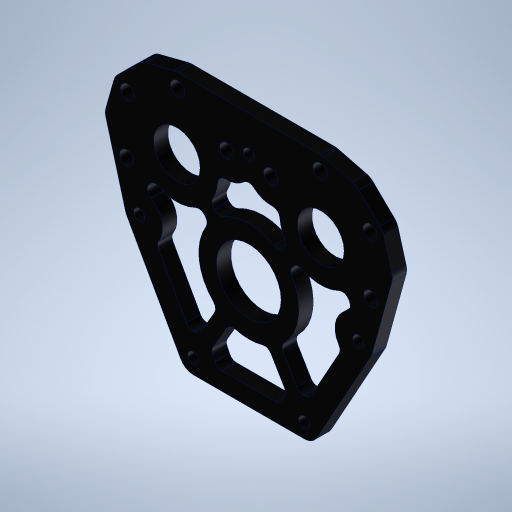
# Autodesk Inventor part: BottomPlate_Gearboxes_2_Exercise_2
Saved by Autodesk Inventor 2024 (Build 280153000, 153)
## iProperties
Created: 2024-11-16
Part Number: BottomPlate_Gearboxes_2_Exercise_2
Material: Aluminum 6061
Document SubType Name: Modeling
Designer: Danielle
Density: 2.7 g/cm^3
Appearance: Aluminum - Flat
Author: Danielle
Autodesk Inventor part; units mm, degrees
ref_plane "YZ Plane" through (0, 0, 0) normal (1, 0, 0) x (0, 1, 0)
ref_plane "XZ Plane" through (0, 0, 0) normal (0, 1, 0) x (-1, 0, 0)
ref_plane "XY Plane" through (0, 0, 0) normal (0, 0, 1) x (1, 0, 0)
sketch "Sketch1" plane through (0, 0, 0) normal (0, 0, 1) x (1, 0, 0)
  circle A0 centre (0, 0) radius 38.1 construction
  circle A1 centre (0, 0) radius 40.64 construction
  circle A2 centre (0, 0) radius 14.2875
  circle A3 centre (-31.9157, 32.7369) radius 30.0609 construction
  circle A4 centre (-31.9157, 32.7369) radius 25.4 construction
  circle A5 centre (-31.9157, 32.7369) radius 7.62 construction
  circle A6 centre (-53.7497, 45.7153) radius 3.175
  circle A7 centre (-57.3137, 33.0595) radius 3.175 construction
  circle A8 centre (-54.0723, 20.3173) radius 3.175
  circle A9 centre (-44.8941, 10.903) radius 3.175 construction
  circle A10 centre (-32.2383, 7.339) radius 3.175 construction
  circle A11 centre (-19.4961, 10.5803) radius 3.175 construction
  circle A12 centre (-10.0817, 19.7586) radius 3.175 construction
  circle A13 centre (-6.5178, 32.4143) radius 3.175 construction
  circle A14 centre (-9.7591, 45.1565) radius 3.175
  circle A15 centre (-18.9373, 54.5709) radius 3.175 construction
  circle A16 centre (-31.5931, 58.1349) radius 3.175
  circle A17 centre (-44.3353, 54.8935) radius 3.175 construction
  line L0 (-54.0723, 20.3173) -> (0, 0) construction
  line L1 (0, 0) -> (-18.9373, 54.5709) construction
  circle A18 centre (-48.5745, 1.2342) radius 2.4892
  circle A19 centre (-48.5745, 1.2342) radius 6.35 construction
  circle A20 centre (-48.5745, 1.2342) radius 3.9751 construction
  line L2 (-46.7163, 4.7482) -> (-45.9682, 6.1628) construction
  line L3 (-42.2266, 1.0729) -> (-40.6269, 1.0322) construction
  circle A21 centre (0, 48.5902) radius 6.35 construction
  circle A22 centre (0, 48.5902) radius 3.9751 construction
  circle A23 centre (0, 48.5902) radius 2.4892
  line L4 (0, 42.2402) -> (0, 40.64) construction
  line L5 (-3.5601, 46.8218) -> (-4.9932, 46.1099) construction
  circle A24 centre (-24.6505, -41.8731) radius 6.35 construction
  circle A25 centre (-24.6505, -41.8731) radius 2.4892
  line L6 (-21.4291, -36.4009) -> (-20.6173, -35.022)
  line L7 (0, 48.5902) -> (0, 0) construction
  circle A26 centre (31.9157, 32.7369) radius 30.0609 construction
  circle A27 centre (31.9157, 32.7369) radius 25.4 construction
  circle A28 centre (53.7497, 45.7153) radius 3.175
  circle A29 centre (57.3137, 33.0595) radius 3.175 construction
  circle A30 centre (54.0723, 20.3173) radius 3.175
  circle A31 centre (44.8941, 10.903) radius 3.175 construction
  circle A32 centre (9.7591, 45.1565) radius 3.175
  circle A33 centre (18.9373, 54.5709) radius 3.175 construction
  circle A34 centre (31.5931, 58.1349) radius 3.175
  circle A35 centre (44.3353, 54.8935) radius 3.175 construction
  circle A36 centre (48.5745, 1.2342) radius 2.4892
  circle A37 centre (48.5745, 1.2342) radius 6.35 construction
  circle A38 centre (48.5745, 1.2342) radius 3.9751 construction
  circle A39 centre (0, 48.5902) radius 2.4892 construction
  circle A40 centre (24.6505, -41.8731) radius 6.35 construction
  circle A41 centre (24.6505, -41.8731) radius 2.4892
  circle A42 centre (31.9157, 32.7369) radius 7.62 construction
  line L8 (-48.5745, 1.2342) -> (-24.6505, -41.8731) construction
  line L9 (24.6505, -41.8731) -> (-24.6505, -41.8731) construction
  circle A43 centre (-31.9157, 32.7369) radius 10.3188
  circle A44 centre (31.9157, 32.7369) radius 10.3188
  line L10 (-54.1268, -1.8472) -> (-30.2028, -44.9545)
  line L11 (-24.6505, -48.2231) -> (24.6505, -48.2231)
  line L12 (30.2028, -44.9545) -> (54.1268, -1.8472)
  circle A45 centre (44.3353, 54.8935) radius 6.35 construction
  circle A46 centre (53.7497, 45.7153) radius 6.35 construction
  circle A47 centre (31.5931, 58.1349) radius 6.35 construction
  circle A48 centre (57.3137, 33.0595) radius 6.35 construction
  circle A49 centre (54.0723, 20.3173) radius 6.35 construction
  circle A50 centre (-54.0723, 20.3173) radius 6.35 construction
  circle A51 centre (-57.3137, 33.0595) radius 6.35 construction
  circle A52 centre (-53.7497, 45.7153) radius 6.35 construction
  circle A53 centre (-44.3353, 54.8935) radius 6.35 construction
  circle A54 centre (-31.5931, 58.1349) radius 6.35 construction
  line L13 (-63.4259, 34.7808) -> (-59.8619, 47.4366)
  line L14 (-58.1824, 50.2621) -> (-48.768, 59.4403)
  line L15 (-45.9008, 61.0475) -> (-33.1586, 64.2889)
  line L16 (63.4259, 34.7808) -> (59.8619, 47.4366)
  line L17 (58.1824, 50.2621) -> (48.768, 59.4403)
  line L18 (45.9008, 61.0475) -> (33.1586, 64.2889)
  line L19 (-63.437, 31.3781) -> (-54.6979, -0.4473)
  line L20 (63.437, 31.3781) -> (54.6979, -0.4473)
  line L21 (-31.5931, 64.4849) -> (31.5931, 64.4849)
  arc A55 (-30.2028, -44.9545) -> (-24.6505, -48.2231) centre (-24.6505, -41.8731) ccw
  arc A56 (-54.6979, -0.4473) -> (-54.1268, -1.8472) centre (-48.5745, 1.2342) ccw
  arc A57 (-63.4259, 34.7808) -> (-63.437, 31.3781) centre (-57.3137, 33.0595) ccw
  arc A58 (-58.1824, 50.2621) -> (-59.8619, 47.4366) centre (-53.7497, 45.7153) ccw
  arc A59 (-45.9008, 61.0475) -> (-48.768, 59.4403) centre (-44.3353, 54.8935) ccw
  arc A60 (-31.5931, 64.4849) -> (-33.1586, 64.2889) centre (-31.5931, 58.1349) ccw
  arc A61 (33.1586, 64.2889) -> (31.5931, 64.4849) centre (31.5931, 58.1349) ccw
  arc A62 (48.768, 59.4403) -> (45.9008, 61.0475) centre (44.3353, 54.8935) ccw
  arc A63 (59.8619, 47.4366) -> (58.1824, 50.2621) centre (53.7497, 45.7153) ccw
  arc A64 (63.437, 31.3781) -> (63.4259, 34.7808) centre (57.3137, 33.0595) ccw
  arc A65 (54.1268, -1.8472) -> (54.6979, -0.4473) centre (48.5745, 1.2342) ccw
  arc A66 (24.6505, -48.2231) -> (30.2028, -44.9545) centre (24.6505, -41.8731) ccw
  dimension "d4" = 50.8
  dimension "d15" = 7.9502
  dimension "d22" = 12.7
  dimension "d0" = 76.2
  dimension "d1" = 2.54
  dimension "d2" = 28.575
  dimension "d3" = 60.1218
  dimension "d5" = 15.24
  dimension "d6" = 6.35
  dimension "d9" = 360
  dimension "d12" = 12.7
  dimension "d14" = 4.9784
  dimension "d16" = 1.6002
  dimension "d17" = 15.24
  dimension "d18" = 20.6375
  dimension "d19" = 20.6375
  dimension "d20" = 12.7
  dimension "d21" = 12.7
  dimension "d23" = 12.7
  dimension "d24" = 12.7
  dimension "d25" = 12.7
  dimension "d26" = 12.7
  dimension "d27" = 12.7
  dimension "d28" = 12.7
  dimension "d29" = 12.7
  constraints: 60 centre point, 45 point on circle, 44 end point, 25 coincident, 23 symmetric about line, 18 tangent, 10 point on line, 9 concentric, 6 equal length, 3 equal radius, 3 horizontal, 3 vertical, 2 vertical alignment, 63 other
  measures "d0" diameter of A0
  measures "d1" radial gap between concentric circles of A1 A0
  measures "d2" diameter of A2
  measures "d3" diameter of A3
  measures "d5" diameter of A5
  measures "d6" diameter of A6
  measures "d12" diameter of A19
  measures "d14" diameter of A18
  measures "d16" distance of L2.start L2.end
  measures "d17" diameter of A42
  measures "d18" diameter of A43
  measures "d19" diameter of A44
  measures "d20" diameter of A45
  measures "d21" diameter of A46
  measures "d23" diameter of A48
  measures "d24" diameter of A49
  measures "d25" diameter of A50
  measures "d26" diameter of A51
  measures "d27" diameter of A52
  measures "d28" diameter of A53
  measures "d29" diameter of A54
extrude "Extrusion1" add sketch "Sketch1" along normal blind 6.35
sketch "Sketch2" plane through (0, 0, 6.35) normal (0, 0, 1) x (1, 0, 0)
  line L0 (-63.437, 31.3781) -> (-54.6979, -0.4473) construction
  arc A0 (-54.6979, -0.4473) -> (-54.1268, -1.8472) centre (-48.5745, 1.2342) ccw construction
  line L1 (-54.1268, -1.8472) -> (-30.2028, -44.9545) construction
  arc A1 (-30.2028, -44.9545) -> (-24.6505, -48.2231) centre (-24.6505, -41.8731) ccw construction
  line L2 (-24.6505, -48.2231) -> (24.6505, -48.2231) construction
  arc A2 (24.6505, -48.2231) -> (30.2028, -44.9545) centre (24.6505, -41.8731) ccw construction
  line L3 (30.2028, -44.9545) -> (54.1268, -1.8472) construction
  arc A3 (54.1268, -1.8472) -> (54.6979, -0.4473) centre (48.5745, 1.2342) ccw construction
  line L4 (54.6979, -0.4473) -> (63.437, 31.3781) construction
  arc A4 (63.437, 31.3781) -> (63.4259, 34.7808) centre (57.3137, 33.0595) ccw construction
  line L5 (63.4259, 34.7808) -> (59.8619, 47.4366) construction
  arc A5 (59.8619, 47.4366) -> (58.1824, 50.2621) centre (53.7497, 45.7153) ccw construction
  line L6 (58.1824, 50.2621) -> (48.768, 59.4403) construction
  arc A6 (48.768, 59.4403) -> (45.9008, 61.0475) centre (44.3353, 54.8935) ccw construction
  line L7 (45.9008, 61.0475) -> (33.1586, 64.2889) construction
  arc A7 (33.1586, 64.2889) -> (31.5931, 64.4849) centre (31.5931, 58.1349) ccw construction
  line L8 (31.5931, 64.4849) -> (-31.5931, 64.4849) construction
  arc A8 (-31.5931, 64.4849) -> (-33.1586, 64.2889) centre (-31.5931, 58.1349) ccw construction
  line L9 (-33.1586, 64.2889) -> (-45.9008, 61.0475) construction
  arc A9 (-45.9008, 61.0475) -> (-48.768, 59.4403) centre (-44.3353, 54.8935) ccw construction
  line L10 (-48.768, 59.4403) -> (-58.1824, 50.2621) construction
  arc A10 (-58.1824, 50.2621) -> (-59.8619, 47.4366) centre (-53.7497, 45.7153) ccw construction
  line L11 (-59.8619, 47.4366) -> (-63.4259, 34.7808) construction
  arc A11 (-63.4259, 34.7808) -> (-63.437, 31.3781) centre (-57.3137, 33.0595) ccw construction
  circle A12 centre (31.9157, 32.7369) radius 10.3188 construction
  circle A13 centre (24.6505, -41.8731) radius 2.4892 construction
  circle A14 centre (9.7591, 45.1565) radius 3.175 construction
  circle A15 centre (53.7497, 45.7153) radius 3.175 construction
  circle A16 centre (0, 48.5902) radius 2.4892 construction
  circle A17 centre (-48.5745, 1.2342) radius 2.4892 construction
  circle A18 centre (-9.7591, 45.1565) radius 3.175 construction
  circle A19 centre (-53.7497, 45.7153) radius 3.175 construction
  circle A20 centre (0, 0) radius 14.2875 construction
  circle A21 centre (-24.6505, -41.8731) radius 2.4892 construction
  circle A22 centre (48.5745, 1.2342) radius 2.4892 construction
  circle A23 centre (-31.9157, 32.7369) radius 10.3188 construction
  circle A24 centre (31.5931, 58.1349) radius 3.175 construction
  circle A25 centre (54.0723, 20.3173) radius 3.175 construction
  circle A26 centre (-31.5931, 58.1349) radius 3.175 construction
  circle A27 centre (-54.0723, 20.3173) radius 3.175 construction
  circle A28 centre (-31.9157, 32.7369) radius 15.0813 construction
  circle A29 centre (31.9157, 32.7369) radius 15.0813 construction
  circle A30 centre (-31.5931, 58.1349) radius 7.9375 construction
  circle A31 centre (-53.7497, 45.7153) radius 7.9375 construction
  circle A32 centre (-54.0723, 20.3173) radius 7.9375 construction
  circle A33 centre (-9.7591, 45.1565) radius 7.9375 construction
  circle A34 centre (9.7591, 45.1565) radius 7.9375 construction
  circle A35 centre (31.5931, 58.1349) radius 7.9375 construction
  circle A36 centre (53.7497, 45.7153) radius 7.9375 construction
  circle A37 centre (54.0723, 20.3173) radius 7.9375 construction
  circle A38 centre (0, 48.5902) radius 7.2517 construction
  circle A39 centre (48.5745, 1.2342) radius 7.2517 construction
  circle A40 centre (24.6505, -41.8731) radius 7.2517 construction
  circle A41 centre (-24.6505, -41.8731) radius 7.2517 construction
  circle A42 centre (-48.5745, 1.2342) radius 7.2517 construction
  circle A43 centre (0, 0) radius 19.05 construction
  line L12 (-26.0386, -42.6435) -> (-49.9626, 0.4638) construction
  arc A44 (-50.1054, 0.8138) -> (-49.9626, 0.4638) centre (-48.5745, 1.2342) ccw construction
  line L13 (-50.1054, 0.8138) -> (-58.8445, 32.6392) construction
  arc A45 (-58.8417, 33.4898) -> (-58.8445, 32.6392) centre (-57.3137, 33.0595) ccw construction
  line L14 (-58.8417, 33.4898) -> (-55.2777, 46.1456) construction
  arc A46 (-54.8579, 46.852) -> (-55.2777, 46.1456) centre (-53.7497, 45.7153) ccw construction
  line L15 (-54.8579, 46.852) -> (-45.4435, 56.0302) construction
  arc A47 (-44.7267, 56.432) -> (-45.4435, 56.0302) centre (-44.3353, 54.8935) ccw construction
  line L16 (-44.7267, 56.432) -> (-31.9845, 59.6734) construction
  arc A48 (-31.5931, 59.7224) -> (-31.9845, 59.6734) centre (-31.5931, 58.1349) ccw construction
  line L17 (-31.5931, 59.7224) -> (31.5931, 59.7224) construction
  arc A49 (31.9845, 59.6734) -> (31.5931, 59.7224) centre (31.5931, 58.1349) ccw construction
  line L18 (31.9845, 59.6734) -> (44.7267, 56.432) construction
  arc A50 (45.4435, 56.0302) -> (44.7267, 56.432) centre (44.3353, 54.8935) ccw construction
  line L19 (45.4435, 56.0302) -> (54.8579, 46.852) construction
  arc A51 (55.2777, 46.1456) -> (54.8579, 46.852) centre (53.7497, 45.7153) ccw construction
  line L20 (55.2777, 46.1456) -> (58.8417, 33.4898) construction
  arc A52 (58.8445, 32.6392) -> (58.8417, 33.4898) centre (57.3137, 33.0595) ccw construction
  line L21 (58.8445, 32.6392) -> (50.1054, 0.8138) construction
  arc A53 (49.9626, 0.4638) -> (50.1054, 0.8138) centre (48.5745, 1.2342) ccw construction
  line L22 (49.9626, 0.4638) -> (26.0386, -42.6435) construction
  arc A54 (24.6505, -43.4606) -> (26.0386, -42.6435) centre (24.6505, -41.8731) ccw construction
  line L23 (24.6505, -43.4606) -> (-24.6505, -43.4606) construction
  arc A55 (-26.0386, -42.6435) -> (-24.6505, -43.4606) centre (-24.6505, -41.8731) ccw construction
  line L24 (-53.7497, 45.7153) -> (-31.9157, 32.7369) construction
  line L25 (-31.9157, 32.7369) -> (0, 0) construction
  line L26 (0, 0) -> (24.6505, -41.8731) construction
  line L27 (-31.5931, 58.1349) -> (-9.7591, 45.1565) construction
  line L28 (-9.7591, 45.1565) -> (0, 48.5902) construction
  line L29 (0, 48.5902) -> (9.7591, 45.1565) construction
  line L30 (9.7591, 45.1565) -> (31.9157, 32.7369) construction
  line L31 (31.9157, 32.7369) -> (53.7497, 45.7153) construction
  line L32 (9.7591, 45.1565) -> (31.5931, 58.1349) construction
  line L33 (31.9157, 32.7369) -> (54.0723, 20.3173) construction
  line L34 (31.9157, 32.7369) -> (0, 0) construction
  line L35 (-24.6505, -41.8731) -> (0, 0) construction
  line L36 (-53.7497, 45.7153) -> (-54.0723, 20.3173) construction
  line L37 (-54.0723, 20.3173) -> (-31.9157, 32.7369) construction
  line L38 (-31.9157, 32.7369) -> (-9.7591, 45.1565) construction
  line L39 (-48.5745, 1.2342) -> (-54.0723, 20.3173) construction
  line L40 (-31.5931, 58.1349) -> (-53.7497, 45.7153) construction
  line L41 (31.5931, 58.1349) -> (53.7497, 45.7153) construction
  line L42 (-24.6505, -41.8731) -> (-48.5745, 1.2342) construction
  line L43 (48.5745, 1.2342) -> (24.6505, -41.8731) construction
  line L44 (48.5745, 1.2342) -> (54.0723, 20.3173) construction
  line L45 (-52.1274, 48.4445) -> (-30.2934, 35.4662)
  line L46 (-8.4463, 42.2526) -> (0, 45.2244)
  line L47 (0, 45.2244) -> (8.4463, 42.2526)
  line L48 (8.4463, 42.2526) -> (26.7539, 31.9905)
  line L49 (26.7539, 31.9905) -> (-2.5414, 1.9415)
  line L50 (-2.5414, 1.9415) -> (-24.5693, -35.4767)
  line L51 (-24.5693, -35.4767) -> (-45.6234, 2.4596)
  line L52 (-45.6234, 2.4596) -> (-50.3247, 18.7782)
  line L53 (-50.3247, 18.7782) -> (-30.3633, 29.9674)
  line L54 (-30.3633, 29.9674) -> (-8.4463, 42.2526)
  line L55 (-11.072, 48.0604) -> (0, 51.956)
  line L56 (0, 51.956) -> (11.072, 48.0604)
  line L57 (11.072, 48.0604) -> (37.0775, 33.4833)
  line L58 (37.0775, 33.4833) -> (2.5414, -1.9415)
  line L59 (2.5414, -1.9415) -> (-24.7318, -48.2696)
  line L60 (-24.7318, -48.2696) -> (-51.5256, 0.0087)
  line L61 (-51.5256, 0.0087) -> (-57.8198, 21.8565)
  line L62 (-57.8198, 21.8565) -> (-33.4682, 35.5065)
  line L63 (-33.4682, 35.5065) -> (-11.072, 48.0604)
  line L64 (-55.372, 42.986) -> (-33.538, 30.0077)
  line L65 (-30.0407, 55.3653) -> (-50.5982, 43.842)
  line L66 (-50.5982, 43.842) -> (-50.8277, 25.7758)
  line L67 (-50.8277, 25.7758) -> (-33.4682, 35.5065)
  line L68 (-33.4682, 35.5065) -> (-11.3116, 47.9261)
  line L69 (-33.2154, 55.4056) -> (-11.3814, 42.4273)
  line L70 (-33.1456, 60.9044) -> (-56.9011, 47.5885)
  line L71 (-56.9011, 47.5885) -> (-57.3169, 14.8588)
  line L72 (-57.3169, 14.8588) -> (-30.3633, 29.9674)
  line L73 (-30.3633, 29.9674) -> (-8.2067, 42.3869)
  line L74 (-29.9708, 60.8641) -> (-8.1368, 47.8858)
  line L75 (-3.9666, -0.4796) -> (-32.4884, 28.7761)
  line L76 (-32.4884, 28.7761) -> (-50.3247, 18.7782)
  line L77 (-50.3247, 18.7782) -> (-45.6234, 2.4596)
  line L78 (-45.6234, 2.4596) -> (-24.5693, -35.4767)
  line L79 (-24.5693, -35.4767) -> (-3.9666, -0.4796)
  line L80 (3.9666, 0.4796) -> (-31.343, 36.6977)
  line L81 (-31.343, 36.6977) -> (-57.8198, 21.8565)
  line L82 (-57.8198, 21.8565) -> (-51.5256, 0.0087)
  line L83 (-51.5256, 0.0087) -> (-24.7318, -48.2696)
  line L84 (-24.7318, -48.2696) -> (3.9666, 0.4796)
  line L85 (31.6397, 54.469) -> (16.1086, 45.2372)
  line L86 (16.1086, 45.2372) -> (31.8691, 36.4028)
  line L87 (31.8691, 36.4028) -> (47.4002, 45.6346)
  line L88 (47.4002, 45.6346) -> (31.6397, 54.469)
  line L89 (60.0992, 45.7959) -> (31.9623, 29.071)
  line L90 (31.9623, 29.071) -> (3.4096, 45.0759)
  line L91 (3.4096, 45.0759) -> (31.5465, 61.8008)
  line L92 (31.5465, 61.8008) -> (60.0992, 45.7959)
  line L93 (57.8198, 21.8565) -> (31.343, 36.6977)
  line L94 (31.343, 36.6977) -> (-3.9666, 0.4796)
  line L95 (-3.9666, 0.4796) -> (24.7318, -48.2696)
  line L96 (24.7318, -48.2696) -> (51.5256, 0.0087)
  line L97 (51.5256, 0.0087) -> (57.8198, 21.8565)
  line L98 (50.3247, 18.7782) -> (32.4884, 28.7761)
  line L99 (32.4884, 28.7761) -> (3.9666, -0.4796)
  line L100 (3.9666, -0.4796) -> (24.5693, -35.4767)
  line L101 (24.5693, -35.4767) -> (45.6234, 2.4596)
  line L102 (45.6234, 2.4596) -> (50.3247, 18.7782)
  line L103 (-23.716, -40.2856) -> (23.716, -40.2856)
  line L104 (23.716, -40.2856) -> (47.0941, 1.8381)
  line L105 (47.0941, 1.8381) -> (55.6659, 33.0542)
  line L106 (55.6659, 33.0542) -> (52.3369, 44.8755)
  line L107 (52.3369, 44.8755) -> (43.5317, 53.4599)
  line L108 (43.5317, 53.4599) -> (31.3944, 56.5474)
  line L109 (31.3944, 56.5474) -> (-31.3944, 56.5474)
  line L110 (-31.3944, 56.5474) -> (-43.5317, 53.4599)
  line L111 (-43.5317, 53.4599) -> (-52.3369, 44.8755)
  line L112 (-52.3369, 44.8755) -> (-55.6659, 33.0542)
  line L113 (-55.6659, 33.0542) -> (-47.0941, 1.8381)
  line L114 (-47.0941, 1.8381) -> (-23.716, -40.2856)
  circle A56 centre (-9.7591, 45.1565) radius 11.1125
  circle A57 centre (0, 48.5902) radius 10.4267
  circle A58 centre (9.7591, 45.1565) radius 11.1125
  circle A59 centre (31.9157, 32.7369) radius 18.2563
  circle A60 centre (0, 0) radius 22.225
  circle A61 centre (-31.9157, 32.7369) radius 18.2563
  circle A62 centre (-24.6505, -41.8731) radius 10.4267
  circle A63 centre (24.6505, -41.8731) radius 10.4267
  circle A64 centre (48.5745, 1.2342) radius 10.4267
  circle A65 centre (54.0723, 20.3173) radius 11.1125
  circle A66 centre (53.7497, 45.7153) radius 11.1125
  circle A67 centre (31.5931, 58.1349) radius 11.1125
  circle A68 centre (-31.5931, 58.1349) radius 11.1125
  circle A69 centre (-53.7497, 45.7153) radius 11.1125
  circle A70 centre (-54.0723, 20.3173) radius 11.1125
  circle A71 centre (-48.5745, 1.2342) radius 10.4267
  point P0 (-13.7759, 34.7954)
  point P1 (-17.0924, 22.0805)
  point P2 (-13.0821, 17.9669)
  point P3 (13.0821, 17.9669)
  point P4 (17.0924, 22.0805)
  point P5 (13.7759, 34.7954)
  point P6 (1.0779, 38.2194)
  point P7 (-1.0779, 38.2194)
  point P8 (47.2161, 11.572)
  point P9 (43.1377, 18.337)
  point P10 (21.6392, 17.6477)
  point P11 (17.6288, 13.5342)
  point P12 (13.8955, -17.3455)
  point P13 (22.3482, -31.7038)
  point P14 (26.6938, -31.6486)
  point P15 (40.979, -5.9089)
  point P16 (14.3454, -40.2856)
  point P17 (16.876, -34.9252)
  point P18 (8.4233, -20.5669)
  point P19 (-8.4233, -20.5669)
  point P20 (-16.876, -34.9252)
  point P21 (-14.3454, -40.2856)
  point P22 (-47.2161, 11.572)
  point P23 (-40.979, -5.9089)
  point P24 (-26.6938, -31.6486)
  point P25 (-22.3482, -31.7038)
  point P26 (-13.8955, -17.3455)
  point P27 (-17.6288, 13.5342)
  point P28 (-21.6392, 17.6477)
  point P29 (-43.1377, 18.337)
  dimension "d32" = 4.7625
  dimension "d33" = 4.7625
  dimension "d34" = 4.7625
  dimension "d35" = 4.7625
  dimension "d36" = 4.7625
  dimension "d37" = 3.175
  dimension "d38" = 3.175
  dimension "d39" = 3.175
  dimension "d40" = 3.175
  dimension "d41" = 3.175
  dimension "d42" = 3.175
  dimension "d43" = 3.175
  dimension "d44" = 3.175
  dimension "d45" = 3.175
  dimension "d46" = 3.175
  dimension "d47" = 3.175
  dimension "d48" = 3.175
  dimension "d49" = 3.175
  dimension "d50" = 3.175
  dimension "d51" = 3.175
  dimension "d52" = 3.175
  dimension "d53" = 3.175
  dimension "d54" = 3.175
  dimension "d55" = 3.175
  dimension "d56" = 3.175
  dimension "d57" = 3.175
  dimension "d58" = 3.175
  dimension "d59" = 3.175
  dimension "d60" = 3.175
  dimension "d61" = 3.175
  dimension "d62" = 3.175
  dimension "d63" = 3.175
  dimension "d64" = 3.175
  dimension "d65" = 3.175
  dimension "d66" = 3.175
  dimension "d67" = 3.175
  constraints: 206 end point, 44 centre point, 24 point on circle, 12 equal radius, 6 parallel, 5 collinear, 1 coincident, 78 other
  measures "d32" radial gap between concentric circles of A23 A28
  measures "d33" radial gap between concentric circles of A26 A30
  measures "d34" radial gap between concentric circles of A16 A38
  measures "d35" radial gap between concentric circles of A20 A43
  measures "d36" distance between parallel lines of L1 L12
  measures "d37" distance between parallel lines of L24 L45
  measures "d38" distance between parallel lines of L38 L54
  measures "d39" distance between parallel lines of L38 L63
  measures "d40" distance between parallel lines of L24 L64
  measures "d41" distance between parallel lines of L40 L65
  measures "d42" distance between parallel lines of L27 L69
  measures "d43" distance between parallel lines of L40 L70
  measures "d44" distance between parallel lines of L27 L74
  measures "d45" distance between parallel lines of L25 L75
  measures "d46" distance between parallel lines of L25 L80
  measures "d47" distance between parallel lines of L32 L85
  measures "d48" distance between parallel lines of L41 L92
  measures "d49" distance between parallel lines of L33 L93
  measures "d50" distance between parallel lines of L33 L98
  measures "d51" distance between parallel lines of L23 L103
  measures "d52" radial gap between concentric circles of A33 A56
  measures "d53" radial gap between concentric circles of A38 A57
  measures "d54" radial gap between concentric circles of A34 A58
  measures "d55" radial gap between concentric circles of A29 A59
  measures "d56" radial gap between concentric circles of A43 A60
  measures "d57" radial gap between concentric circles of A28 A61
  measures "d58" radial gap between concentric circles of A41 A62
  measures "d59" radial gap between concentric circles of A40 A63
  measures "d60" radial gap between concentric circles of A39 A64
  measures "d61" radial gap between concentric circles of A37 A65
  measures "d62" radial gap between concentric circles of A36 A66
  measures "d63" radial gap between concentric circles of A35 A67
  measures "d64" radial gap between concentric circles of A30 A68
  measures "d65" radial gap between concentric circles of A31 A69
  measures "d66" radial gap between concentric circles of A32 A70
  measures "d67" radial gap between concentric circles of A42 A71
extrude "Extrusion2" cut sketch "Sketch2" against normal blind 25.4 contours A61 A56 A57 A58 A59 L49 A60 L80 | L75 A60 L50 A62 L51 A71 A70 A61 | A62 L59 A60 L95 A63 L103 | L58 A59 A65 A64 L101 A63 L100 A60
fillet "Fillet1" radius 3.175 1 edges at (13.8955, -17.3455, 3.175)
fillet "Fillet2" radius 3.175 7 edges at (17.6288, 13.5342, 3.175) (21.6392, 17.6477, 3.175) (43.1377, 18.337, 3.175) (47.2161, 11.572, 3.175) (40.979, -5.9089, 3.175) (26.6938, -31.6486, 3.175) (22.3482, -31.7038, 3.175)
fillet "Fillet3" radius 3.175 6 edges at (-8.4233, -20.5669, 3.175) (8.4233, -20.5669, 3.175) (-16.876, -34.9252, 3.175) (-14.3454, -40.2856, 3.175) (14.3454, -40.2856, 3.175) (16.876, -34.9252, 3.175)
fillet "Fillet4" radius 3.175 8 edges at (-26.6938, -31.6486, 3.175) (-22.3482, -31.7038, 3.175) (-40.979, -5.9089, 3.175) (-47.2161, 11.572, 3.175) (-43.1377, 18.337, 3.175) (-21.6392, 17.6477, 3.175) (-17.6288, 13.5342, 3.175) (-13.8955, -17.3455, 3.175)
fillet "Fillet5" radius 3.175 8 edges at (-1.0779, 38.2194, 3.175) (1.0779, 38.2194, 3.175) (13.7759, 34.7954, 3.175) (17.0924, 22.0805, 3.175) (13.0821, 17.9669, 3.175) (-13.0821, 17.9669, 3.175) (-17.0924, 22.0805, 3.175) (-13.7759, 34.7954, 3.175)
body "Solid1"
